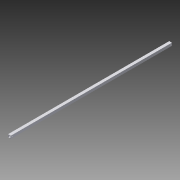
# Autodesk Inventor part: NTowerSupport
Saved by Autodesk Inventor 2015 (Build 190159000, 159)
## iProperties
Created: 2015-01-28
Part Number: NTowerSupport
Material: Aluminum 6061
Document SubType Name: Modeling
Designer: Andrew
Density: 2.7 g/cm^3
Appearance: Aluminum - Flat
Author: Andrew
Autodesk Inventor part; units mm, degrees
ref_plane "YZ Plane" through (0, 0, 0) normal (1, 0, 0) x (0, 1, 0)
ref_plane "XZ Plane" through (0, 0, 0) normal (0, 1, 0) x (-1, 0, 0)
ref_plane "XY Plane" through (0, 0, 0) normal (0, 0, 1) x (1, 0, 0)
sketch "Sketch1" plane through (0, 0, 0) normal (0, 0, 1) x (1, 0, 0)
  line L0 (-12.7, 12.7) -> (12.7, 12.7)
  line L1 (12.7, 12.7) -> (12.7, -12.7)
  line L2 (12.7, -12.7) -> (-12.7, -12.7)
  line L3 (-12.7, -12.7) -> (-12.7, 12.7)
  line L4 (0, 17.78) -> (0, -17.78) projected
  line L5 (-17.78, 0) -> (17.78, 0) projected
  line L6 (9.525, 9.525) -> (-9.525, 9.525)
  line L7 (-9.525, 9.525) -> (-9.525, -9.525)
  line L8 (-9.525, -9.525) -> (9.525, -9.525)
  line L9 (9.525, -9.525) -> (9.525, 9.525)
  point P0 (0, 0)
  dimension "d0" = 25.4
  dimension "d1" = 3.175
  constraints: 16 end point, 4 parallel, 3 perpendicular, 1 horizontal, 5 other
  measures "d0" distance of L0.end L1.end
  measures "d1" distance between parallel lines of L0 L6
extrude "Extrusion1" add sketch "Sketch1" along normal mid plane 1502.0343 contours L0 L4 L6 L7 L5 L3 | L0 L1 L5 L9 L6 L4 | L5 L7 L8 L4 L2 L3 | L1 L2 L4 L8 L9 L5
sketch "Sketch2" plane through (12.7, 12.7, 751.0172) normal (1, 0, 0) x (0, 0, -1)
  line L0 (-300.4069, -12.7) -> (1802.4412, -12.7) projected
  line L1 (751.0172, -30.48) -> (751.0172, 5.08) projected
  circle A0 centre (12.7, -12.7) radius 3.175
  circle A1 centre (1489.3343, -12.7) radius 3.175
  point P0 (751.0172, -12.7)
  dimension "d4" = 1476.6343
  dimension "d5" = 6.35
  constraints: 2 centre point, 2 point on line, 1 other
  measures "d4" distance of A1.centre A0.centre
  measures "d5" diameter of A1
extrude "Extrusion2" cut sketch "Sketch2" against normal up to surface (25.4 mm away)
equation "\"d2\" = Length"
equation "\"d6\" = Length"
equation "\"Length\" = 1502.034303"
body "Solid1"
